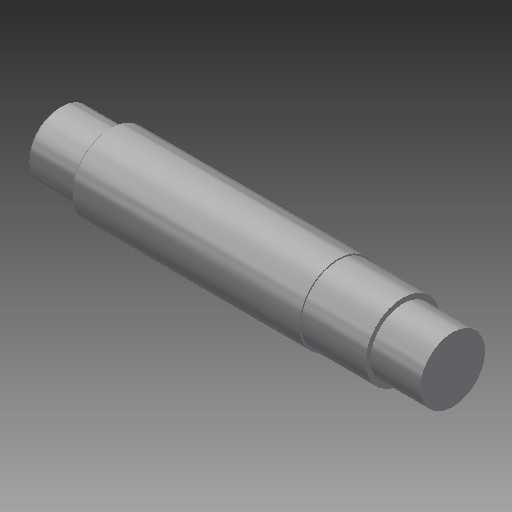
# Autodesk Inventor part: Pedales - Eje
Saved by Autodesk Inventor 2019 (Build 230136000, 136)
## iProperties
Created: 2019-11-15
Part Number: Pedales - Eje
Material: Steel
Document SubType Name: Modeling
Designer: Sanoli
Density: 1 g/cm^3
Appearance: Steel
CustomPartVersion: 1
Author: Sanoli
Autodesk Inventor part; units mm, degrees
ref_plane "Start Plane" through (0, 0, 0) normal (1, 0, 0) x (0, 1, 0)
ref_plane "XZ Plane" through (0, 0, 0) normal (0, 1, 0) x (-1, 0, 0)
ref_plane "XY Plane" through (0, 0, 0) normal (0, 0, 1) x (1, 0, 0)
sketch "Main Sketch" plane through (0, 0, 0) normal (0, 0, 1) x (1, 0, 0)
  line L0 (0, 0) -> (79, 0)
  line L1 (0, 0) -> (0, 6.5)
  line L2 (0, 6.5) -> (10, 6.5)
  line L3 (10, 6.5) -> (10, 7.8)
  line L4 (56, 7.8) -> (56, 7.5)
  line L5 (10, 7.8) -> (56, 7.8)
  line L6 (69, 7.5) -> (69, 6.5)
  line L7 (56, 7.5) -> (69, 7.5)
  line L8 (79, 6.5) -> (79, 0)
  line L9 (69, 6.5) -> (79, 6.5)
  dimension "d3" = 13
  dimension "d4" = 15.6
  dimension "d5" = 15
  dimension "d6" = 13
  constraints: 20 end point, 5 vertical, 1 horizontal
  measures "d3" diameter of L2 L0
  measures "d4" diameter of L5 L0
  measures "d5" diameter of L7 L0
  measures "d6" diameter of L9 L0
revolve "Revolution1" add sketch "Main Sketch" angle 360 about axis through (0, 0, 0) along (1, 0, 0)
chamfer "Chamfer4" distance 0.5 angle 45 1 edges at (0, -6.5, 0) measured on face at (3.3333, 6.4158, -1.0427)
chamfer "Chamfer2" distance 0.5 angle 45 1 edges at (10, -6.5, 0) measured on face at (3.6667, 6.4789, -0.523)
chamfer "Chamfer3" distance 0.5 angle 45 1 edges at (10, -7.8, 0) measured on face at (25.3333, 7.699, -1.2512)
body "Solid1"
